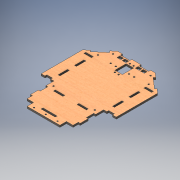
# Autodesk Inventor part: base
Saved by Autodesk Inventor 2019 (Build 230136000, 136)
## iProperties
Created: 2020-12-06
Part Number: base
Material: Дерево (береза)
Document SubType Name: Modeling
Designer: Professional
Density: 0.55 g/cm^3
Appearance: Береза — натуральный — полированный
Author: Professional
Autodesk Inventor part; units mm, degrees
ref_plane "YZ Plane" through (0, 0, 0) normal (1, 0, 0) x (0, 1, 0)
ref_plane "XZ Plane" through (0, 0, 0) normal (0, 1, 0) x (-1, 0, 0)
ref_plane "XY Plane" through (0, 0, 0) normal (0, 0, 1) x (1, 0, 0)
sketch "Эскиз1" plane through (0, 0, 0) normal (0, 1, 0) x (-1, 0, 0)
  line L0 (40, -188.2) -> (80, -153.2) construction
  line L1 (80, -153.2) -> (80, -65.2) construction
  line L2 (0, -188.2) -> (0, 0)
  line L3 (80, -65.2) -> (53, -65.2) construction
  line L4 (53, -65.2) -> (53, 0) construction
  line L5 (40, -188.2) -> (0, -188.2) construction
  line L6 (53, 0) -> (0, 0) construction
  line L7 (49, -15.2) -> (53, -15.2)
  line L8 (53, -15.2) -> (53, -32.2)
  line L9 (53, -32.2) -> (49, -32.2)
  line L10 (49, -32.2) -> (49, -48.2)
  line L11 (49, -48.2) -> (53, -48.2)
  line L12 (60, -65.2) -> (60, -69.2)
  line L13 (60, -69.2) -> (72, -69.2)
  line L14 (72, -69.2) -> (72, -65.2)
  line L15 (72, -65.2) -> (80, -65.2)
  line L16 (80, -65.2) -> (80, -153.2)
  line L17 (80, -153.2) -> (70.9691, -161.1021)
  line L18 (70.9691, -161.1021) -> (68.3351, -158.0917)
  line L19 (46.3969, -177.2876) -> (49.0309, -180.2979)
  line L20 (49.0309, -180.2979) -> (40, -188.2)
  line L21 (40, -188.2) -> (30, -188.2)
  line L22 (30, -188.2) -> (30, -184.2)
  line L23 (30, -184.2) -> (10, -184.2)
  line L24 (10, -184.2) -> (10, -188.2)
  line L25 (-40, -188.2) -> (-80, -153.2) construction
  line L26 (-80, -153.2) -> (-80, -65.2) construction
  line L27 (-80, -65.2) -> (-53, -65.2) construction
  line L28 (-53, -65.2) -> (-53, 0) construction
  line L29 (-40, -188.2) -> (0, -188.2) construction
  line L30 (-53, 0) -> (0, 0) construction
  line L31 (-49, -15.2) -> (-53, -15.2)
  line L32 (-53, -15.2) -> (-53, -32.2)
  line L33 (-53, -32.2) -> (-49, -32.2)
  line L34 (-49, -32.2) -> (-49, -48.2)
  line L35 (-49, -48.2) -> (-53, -48.2)
  line L36 (-60, -65.2) -> (-60, -69.2)
  line L37 (-60, -69.2) -> (-72, -69.2)
  line L38 (-72, -69.2) -> (-72, -65.2)
  line L39 (-72, -65.2) -> (-80, -65.2)
  line L40 (-80, -65.2) -> (-80, -153.2)
  line L41 (-40, -188.2) -> (-30, -188.2)
  line L42 (-30, -188.2) -> (-30, -184.2)
  line L43 (-30, -184.2) -> (-10, -184.2)
  line L44 (-10, -184.2) -> (-10, -188.2)
  line L45 (-10, -188.2) -> (10, -188.2)
  line L46 (68.3351, -158.0917) -> (46.3969, -177.2876)
  line L47 (-80, -153.2) -> (-70.9691, -161.1021)
  line L48 (-70.9691, -161.1021) -> (-68.3351, -158.0917)
  line L49 (-46.3969, -177.2876) -> (-49.0309, -180.2979)
  line L50 (-49.0309, -180.2979) -> (-40, -188.2)
  line L51 (-68.3351, -158.0917) -> (-46.3969, -177.2876)
  line L52 (60, -81.2) -> (56, -81.2)
  line L53 (56, -81.2) -> (56, -101.2)
  line L54 (56, -101.2) -> (60, -101.2)
  line L55 (60, -101.2) -> (60, -81.2)
  line L56 (60, -116.2) -> (56, -116.2)
  line L57 (56, -116.2) -> (56, -136.2)
  line L58 (56, -136.2) -> (60, -136.2)
  line L59 (60, -136.2) -> (60, -116.2)
  line L60 (72, -148.2) -> (56, -148.2)
  line L61 (56, -148.2) -> (56, -152.2)
  line L62 (56, -152.2) -> (72, -152.2)
  line L63 (72, -152.2) -> (72, -148.2)
  line L64 (-60, -81.2) -> (-56, -81.2)
  line L65 (-56, -81.2) -> (-56, -101.2)
  line L66 (-56, -101.2) -> (-60, -101.2)
  line L67 (-60, -101.2) -> (-60, -81.2)
  line L68 (-60, -116.2) -> (-56, -116.2)
  line L69 (-56, -116.2) -> (-56, -136.2)
  line L70 (-56, -136.2) -> (-60, -136.2)
  line L71 (-60, -136.2) -> (-60, -116.2)
  line L72 (-72, -148.2) -> (-56, -148.2)
  line L73 (-56, -148.2) -> (-56, -152.2)
  line L74 (-56, -152.2) -> (-72, -152.2)
  line L75 (-72, -152.2) -> (-72, -148.2)
  line L76 (40, -188.2) -> (40, -184.2) construction
  line L77 (40, -184.2) -> (30, -184.2) construction
  line L78 (53, -48.2) -> (53, -65.2)
  line L79 (60, -65.2) -> (53, -65.2)
  line L80 (-53, -48.2) -> (-53, -65.2)
  line L81 (-60, -65.2) -> (-53, -65.2)
  line L82 (49, -15.2) -> (49, -4)
  line L83 (49, -4) -> (35, -4)
  line L84 (35, -4) -> (35, 0)
  line L85 (35, 0) -> (15, 0)
  line L86 (15, 0) -> (15, -4)
  line L87 (15, -4) -> (0, -4)
  line L88 (-49, -4) -> (-35, -4)
  line L89 (-35, -4) -> (-35, 0)
  line L90 (-35, 0) -> (-15, 0)
  line L91 (-15, 0) -> (-15, -4)
  line L92 (-15, -4) -> (0, -4)
  line L93 (-49, -4) -> (-49, -15.2)
  line L94 (35, -46.4) -> (15, -46.4)
  line L95 (15, -46.4) -> (15, -50.4)
  line L96 (15, -50.4) -> (35, -50.4)
  line L97 (35, -50.4) -> (35, -46.4)
  line L98 (-15, -46.4) -> (-35, -46.4)
  line L99 (-35, -46.4) -> (-35, -50.4)
  line L100 (-35, -50.4) -> (-15, -50.4)
  line L101 (-15, -50.4) -> (-15, -46.4)
  line L102 (8, -150.2) -> (-8, -150.2)
  line L103 (-8, -150.2) -> (-8, -174.2)
  line L104 (-8, -174.2) -> (8, -174.2)
  line L105 (8, -174.2) -> (8, -150.2)
  line L106 (8, -150.2) -> (-8, -174.2) construction
  line L107 (-8, -150.2) -> (8, -174.2) construction
  point P0 (0, -162.2)
  dimension "d1" = 160
  dimension "d2" = 106
  dimension "d3" = 65.2
  dimension "d5" = 80
  dimension "d6" = 88
  dimension "d7" = 27
  dimension "d14" = 4
  dimension "d15" = 15.2
  dimension "d16" = 16
  dimension "d19" = 17
  dimension "d20" = 12
  dimension "d21" = 8
  dimension "d25" = 12
  dimension "d26" = 12
  dimension "d29" = 20
  dimension "d32" = 10
  dimension "d35" = 20
  dimension "d37" = 29.1507
  dimension "d38" = 20
  dimension "d39" = 20
  dimension "d40" = 15
  dimension "d41" = 12
  dimension "d42" = 16
  dimension "d44" = 12
  dimension "d45" = 8
  dimension "d46" = 1
  dimension "d47" = 17
  dimension "d48" = 35
  dimension "d50" = 20
  dimension "d51" = 30
  dimension "d52" = 14
  dimension "d53" = 20
  dimension "d54" = 30
  dimension "d55" = 46.4
  dimension "d56" = 24
  dimension "d57" = 16
  dimension "d58" = 10
  constraints: 217 end point, 41 symmetric about line, 27 point on line, 20 perpendicular, 13 parallel, 12 equal length, 11 horizontal, 8 vertical, 5 collinear, 2 midpoint, 1 vertical alignment, 2 other
  measures "d1" diameter of L1 L2
  measures "d2" diameter of L4 L2
  measures "d3" distance between parallel lines of L3 L6
  measures "d5" diameter of L0.start L2
  measures "d6" distance of L0.end L1.end
  measures "d7" distance between parallel lines of L1 L4
  measures "d14" distance of L10.end L11.end
  measures "d15" distance between parallel lines of L6 L7
  measures "d16" distance between parallel lines of L11 L9
  measures "d19" distance between parallel lines of L7 L9
  measures "d20" distance between parallel lines of L14 L12
  measures "d21" distance between parallel lines of L1 L14
  measures "d25" distance from line of L18 L0.end
  measures "d26" distance from line of L19 L0.start
  measures "d29" distance between parallel lines of L22 L24
  measures "d32" distance from line of L0.start L22
  measures "d35" distance between parallel lines of L44 L24
  measures "d37" distance between parallel lines of L19 L18
  measures "d38" distance of L58.end L56.start
  measures "d39" distance between parallel lines of L1 L55
  measures "d40" distance between parallel lines of L54 L56
  measures "d41" distance between parallel lines of L13 L52
  measures "d42" distance of L60.start L60.end
  measures "d44" distance between parallel lines of L58 L60
  measures "d45" distance between parallel lines of L1 L63
  measures "d46" distance from line of L0.end L62
  measures "d47" distance between parallel lines of L11 L3
  measures "d48" distance from line of L21 L0.end
  measures "d50" distance between parallel lines of L86 L84
  measures "d51" diameter of L86 L2
  measures "d52" distance between parallel lines of L82 L84
  measures "d53" distance of L95.end L96.end
  measures "d54" distance between parallel lines of L101 L95
  measures "d55" distance between parallel lines of L94 L85
  measures "d56" distance between parallel lines of L102 L104
  measures "d57" distance between parallel lines of L103 L105
  measures "d58" distance between parallel lines of L23 L104
extrude "Выдавливание1" add sketch "Эскиз1" along normal blind 4 contours L45 L44 L43 L42 L41 L50 L49 L51 L48 L47 L40 L39 L38 L37 L36 L81 L80 L35 L34 L33 L32 L31 L93 L88 L89 L90 L91 L92 L2 L102 L103 L104 | L2 L104 L105 L102 L87 L86 L85 L84 L83 L82 L7 L8 L9 L10 L11 L78 L79 L12 L13 L14 L15 L16 L17 L18 L46 L19 L20 L21 L22 L23 L24 L45
sketch "Эскиз3" plane through (0, 4, 0) normal (0, 1, 0) x (1, 0, 0)
  line L0 (-8, 150.2) -> (-8, 174.2) projected
  line L1 (-8, 162.2) -> (8, 162.2)
  line L2 (8, 174.2) -> (8, 150.2) projected
  line L3 (-8, 174.2) -> (8, 174.2) projected
  line L4 (0, 174.2) -> (0, 158.8523)
  line L5 (-49, 48.2) -> (-49, 32.2) projected
  line L6 (-35, 50.4) -> (-15, 50.4) projected
  line L7 (-30, 188.2) -> (-40, 188.2) projected
  line L8 (-80, 153.2) -> (-80, 65.2) projected
  point P0 (0, 0)
  point P1 (-4, 146.2)
  point P2 (4, 146.2)
  point P3 (-4, 178.2)
  point P4 (4, 178.2)
  point P5 (44, 55.4)
  point P6 (-44, 55.4)
  point P7 (40, 178.2)
  point P8 (54, 160.2)
  point P9 (-40, 178.2)
  point P10 (-54, 160.2)
  dimension "d66" = 8
  dimension "d67" = 32
  dimension "d83" = 5
  dimension "d84" = 5
  dimension "d85" = 10
  dimension "d86" = 28
  dimension "d87" = 26
  dimension "d88" = 40
  constraints: 6 symmetric about line, 4 end point, 3 midpoint, 1 horizontal alignment, 1 vertical
  measures "d66" distance of point (-4, 178.2) point (4, 178.2)
  measures "d67" distance of point (4, 146.2) point (4, 178.2)
  measures "d83" distance from line of L5 point (-44, 55.4)
  measures "d84" distance from line of point (-44, 55.4) L6
  measures "d85" distance from line of L7 point (-40, 178.2)
  measures "d86" distance from line of L7 point (-54, 160.2)
  measures "d87" distance from line of L8 point (-54, 160.2)
  measures "d88" distance from line of L8 point (-40, 178.2)
hole "Отверстие1" at (-4, 4, -146.2) at (4, 4, -146.2) at (-4, 4, -178.2) at (4, 4, -178.2) at (44, 4, -55.4) at (-44, 4, -55.4) at (40, 4, -178.2) at (54, 4, -160.2) at (-40, 4, -178.2) at (-54, 4, -160.2) direction (0, -1, 0) diameter 3 end through all
sketch "Эскиз4" plane through (0, 4, 0) normal (0, 1, 0) x (1, 0, 0)
  line L0 (-10, 175.7) -> (-18, 175.7)
  line L1 (-18, 175.7) -> (-18, 181.7)
  line L2 (-18, 181.7) -> (-10, 181.7)
  line L3 (-10, 181.7) -> (-10, 175.7)
  line L4 (-8, 150.2) -> (-8, 174.2) projected
  line L5 (-10, 184.2) -> (-30, 184.2) projected
  circle A0 centre (-14, 158.2) radius 1.5
  line L6 (-21, 175.7) -> (-29, 175.7)
  line L7 (-29, 175.7) -> (-29, 181.7)
  line L8 (-29, 181.7) -> (-21, 181.7)
  line L9 (-21, 181.7) -> (-21, 175.7)
  circle A1 centre (-25, 158.2) radius 1.5
  line L10 (-8, 150.2) -> (8, 150.2) projected
  line L11 (0, 150.2) -> (0, 174.2)
  line L12 (-8, 174.2) -> (8, 174.2) projected
  line L13 (10, 175.7) -> (18, 175.7)
  line L14 (18, 175.7) -> (18, 181.7)
  line L15 (18, 181.7) -> (10, 181.7)
  line L16 (10, 181.7) -> (10, 175.7)
  circle A2 centre (14, 158.2) radius 1.5
  line L17 (21, 175.7) -> (29, 175.7)
  line L18 (29, 175.7) -> (29, 181.7)
  line L19 (29, 181.7) -> (21, 181.7)
  line L20 (21, 181.7) -> (21, 175.7)
  circle A3 centre (25, 158.2) radius 1.5
  point P0 (0, 0)
  point P1 (-14, 175.7)
  point P2 (-25, 175.7)
  point P3 (14, 175.7)
  point P4 (25, 175.7)
  dimension "d68" = 8
  dimension "d69" = 6
  dimension "d70" = 2
  dimension "d71" = 2.5
  dimension "d72" = 3
  dimension "d73" = 17.5
  dimension "d76" = 11
  constraints: 34 end point, 12 symmetric about line, 4 centre point, 3 midpoint, 2 horizontal, 2 parallel, 1 perpendicular, 1 vertical alignment, 13 other
  measures "d68" distance between parallel lines of L3 L1
  measures "d69" distance between parallel lines of L2 L0
  measures "d70" distance between parallel lines of L3 L4
  measures "d71" distance between parallel lines of L5 L2
  measures "d72" diameter of A0
  measures "d73" distance from line of L0 A0.centre
  measures "d76" distance of L0.start L6.start
extrude "Выдавливание2" cut sketch "Эскиз4" against normal through all contours L0 L1 L2 L3 | A0 | L6 L7 L8 L9 | A1 | L16 L15 L14 L13 | A2 | L20 L19 L18 L17 | A3
sketch "Эскиз5" plane through (0, 4, 0) normal (0, 1, 0) x (1, 0, 0)
  line L0 (-35, 4) -> (-35, 0) projected
  line L1 (-35, 0) -> (35, 0)
  line L2 (35, 0) -> (35, -10)
  line L3 (35, -10) -> (-35, -10)
  line L4 (-35, -10) -> (-35, 0)
  point P0 (0, 0)
  dimension "d89" = 10
  constraints: 8 end point, 2 parallel, 1 coincident, 1 horizontal, 1 perpendicular
  measures "d89" distance between parallel lines of L1 L3
extrude "Выдавливание3" add sketch "Эскиз5" against normal blind 4
sketch "Эскиз6" plane through (0, 4, 0) normal (0, 1, 0) x (1, 0, 0)
  line L0 (35, -10) -> (-35, -10) projected
  line L1 (0, -10) -> (0, 188.2)
  line L2 (10, 188.2) -> (-10, 188.2) projected
  point P0 (0, 0)
  point P1 (-25, -5)
  point P2 (25, -5)
  point P3 (0, -5)
  dimension "d99" = 5
  dimension "d100" = 50
  constraints: 2 end point, 2 horizontal alignment, 2 midpoint, 1 point on line, 1 symmetric about line
  measures "d99" distance from line of L0 point (25, -5)
  measures "d100" distance of point (25, -5) point (-25, -5)
hole "Отверстие2" at (-25, 4, 5) at (25, 4, 5) at (0, 4, 5) direction (0, -1, 0) diameter 2.8 end through all
